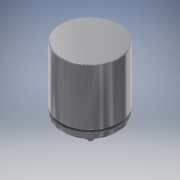
# Autodesk Inventor part: Tachometer
Saved by Autodesk Inventor 2017 (Build 210142000, 142)
## iProperties
Created: 2017-03-05
Part Number: Tachometer
Material: Generic
Document SubType Name: Modeling
Designer: erive
Density: 1 g/cm^3
Appearance: Aluminum - Polished
Author: erive
Autodesk Inventor part; units mm, degrees
ref_plane "YZ Plane" through (0, 0, 0) normal (1, 0, 0) x (0, 1, 0)
ref_plane "XZ Plane" through (0, 0, 0) normal (0, 1, 0) x (-1, 0, 0)
ref_plane "XY Plane" through (0, 0, 0) normal (0, 0, 1) x (1, 0, 0)
sketch "Sketch1" plane through (0, 0, 0) normal (1, 0, 0) x (0, 1, 0)
  line L0 (0, 0) -> (0, 84)
  line L1 (0, 84) -> (29, 84)
  line L2 (29, 84) -> (29, 28)
  line L3 (29, 28) -> (25, 28)
  line L4 (25, 28) -> (25, 25)
  line L5 (25, 25) -> (29, 25)
  line L6 (29, 25) -> (29, 22)
  line L7 (29, 22) -> (25, 22)
  line L8 (25, 22) -> (25, 18)
  line L9 (25, 18) -> (3, 18)
  line L10 (3, 18) -> (3, 0)
  line L11 (3, 0) -> (0, 0)
  dimension "d0" = 84
  dimension "d1" = 29
  dimension "d2" = 56
  dimension "d5" = 4
  dimension "d6" = 3
  dimension "d7" = 4
  dimension "d8" = 3
  dimension "d9" = 4
  dimension "d10" = 4
  dimension "d11" = 22
  constraints: 24 end point, 8 perpendicular, 2 point on line, 1 horizontal, 1 vertical
  measures "d0" distance of L0.start L0.end
  measures "d1" distance of L0.end L1.end
  measures "d2" distance of L1.end L2.end
  measures "d5" distance of L2.end L3.end
  measures "d6" distance of L3.end L4.end
  measures "d7" distance of L4.end L5.end
  measures "d8" distance of L5.end L6.end
  measures "d9" distance of L6.end L7.end
  measures "d10" distance of L7.end L8.end
  measures "d11" distance of L8.end L9.end
revolve "Revolution1" add sketch "Sketch1" angle 360 about axis through (0, 0, 0) along (0, 0, 1)
fillet "Fillet1" radius 1 1 edges at (0, -29, 84)
chamfer "Chamfer1" distance 0.5 angle 45 1 edges at (0, -29, 28)
sketch "Sketch2" plane through (0, 0, 18) normal (0, 0, -1) x (-1, 0, 0)
  line L0 (0, 0) -> (0, -21)
  circle A0 centre (0, -21) radius 1
  circle A1 centre (18.1865, 10.5) radius 1
  circle A2 centre (-18.1865, 10.5) radius 1
  dimension "d17" = 21
  dimension "d18" = 2
  dimension "d21" = 360
  constraints: 3 centre point, 2 end point, 1 coincident, 1 vertical, 7 other
  measures "d17" distance of L0.start L0.end
  measures "d18" diameter of A0
extrude "Extrusion1" cut sketch "Sketch2" against normal blind 8
hole "Hole1" at (0, -21, 18) direction (0, 0, 1) diameter 3.242 depth 11.8 tip angle 118 thread size "M4x0.7" class "6H" standard "ISO Metric profile"
hole "Hole2" at (18.1865, 10.5, 18) direction (0, 0, 1) diameter 3.242 depth 11.8 tip angle 118 thread size "M4x0.7" class "6H" standard "ISO Metric profile"
hole "Hole3" at (-18.1865, 10.5, 18) direction (0, 0, 1) diameter 3.242 depth 11.8 tip angle 118 thread size "M4x0.7" class "6H" standard "ISO Metric profile"
sketch "Sketch5" plane through (0, 0, 0) normal (0, 0, -1) x (-1, 0, 0)
  point P0 (0, 0)
sketch "Sketch6" plane through (0, 0, 0) normal (0, 0, -1) x (-1, 0, 0)
  line L0 (0, 0) -> (0, -3)
  dimension "d62" = 3
  constraints: 2 end point, 1 vertical
  measures "d62" distance of L0.start L0.end
ref_plane "Work Plane2" through (0, -3, 0) normal (0, -1, 0) x (1, 0, 0)
sketch "Sketch7" plane through (0, -3, 0) normal (0, -1, 0) x (1, 0, 0)
  line L0 (-3, 18) -> (-3, 0) projected
  line L1 (3, 18) -> (3, 0) projected
  line L2 (-3, 0) -> (3, 0) projected
  line L3 (-25, 18) -> (25, 18) projected
  line L4 (-1, 0) -> (1, 0)
  line L5 (1, 0) -> (1, 10)
  line L6 (1, 10) -> (-1, 10)
  line L7 (-1, 10) -> (-1, 0)
  point P0 (0, 0)
  dimension "d63" = 10
  dimension "d64" = 2
  dimension "d66" = 2
  constraints: 8 end point, 2 parallel, 1 horizontal, 1 perpendicular, 1 point on line
  measures "d63" distance between parallel lines of L2 L6
  measures "d64" distance between parallel lines of L7 L5
  measures "d66" distance between parallel lines of L0 L7
extrude "Extrusion3" cut sketch "Sketch7" against normal blind 2 contours L7 L6 L5 L2
chamfer "Chamfer3" distance 0.25 angle 45 2 edges at (2.9568, 0.5073, 0) (-2.9568, 0.5073, 0)
body "Solid1"
